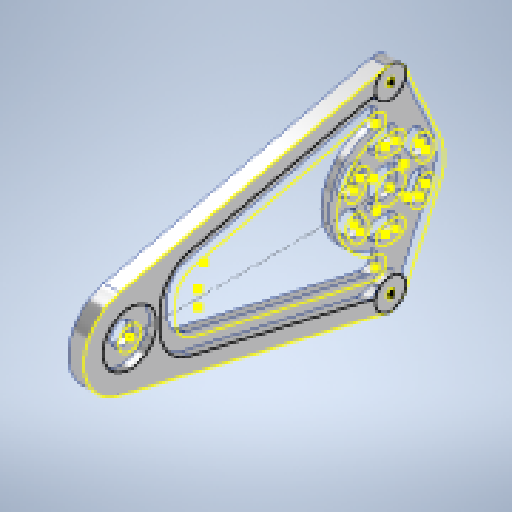
# Autodesk Inventor part: Frame (Motor Side)
Saved by Autodesk Inventor 2023.2 (Build 272271000, 271)
## iProperties
Created: 2022-05-22
Part Number: Frame (Motor Side)
Material: Aluminum 6061
Document SubType Name: Modeling
Designer: Nathan Cai
Density: 2.7 g/cm^3
Appearance: Aluminum - Flat
Mass: 77.655 g
Surface Area: 168.164 cm^2
Volume: 28.7611 cm^3
Author: Nathan Cai
Autodesk Inventor part; units mm, degrees
ref_plane "YZ Plane" through (0, 0, 0) normal (1, 0, 0) x (0, 1, 0)
ref_plane "XZ Plane" through (0, 0, 0) normal (0, 1, 0) x (-1, 0, 0)
ref_plane "XY Plane" through (0, 0, 0) normal (0, 0, 1) x (1, 0, 0)
sketch "Sketch1" plane through (0, 0, 0) normal (1, 0, 0) x (0, 1, 0)
  circle A0 centre (0, 0) radius 6
  circle A1 centre (0, 0) radius 22.225
  line L0 (0, 0) -> (0, 108.331) construction
  circle A2 centre (0, 108.331) radius 4.7625
  circle A3 centre (0, 108.331) radius 76.2 construction
  circle A4 centre (0, 108.331) radius 19.05
  line L1 (0, 0) -> (38.1, 0) construction
  circle A5 centre (38.1, 0) radius 1.7526
  arc A6 (31.9134, -1.4314) -> (35.4542, 5.7725) centre (38.1, 0) ccw
  line L2 (40.7458, -5.7725) -> (9.2604, -20.2038)
  line L3 (18.5597, 112.6252) -> (44.2866, 1.4314)
  line L4 (10.2351, 92.2641) -> (31.9134, -1.4314)
  line L5 (35.4542, 5.7725) -> (22.2231, -0.2919) construction
  circle A7 centre (-38.1, 0) radius 1.7526
  arc A8 (-35.4542, 5.7725) -> (-31.9134, -1.4314) centre (-38.1, 0) ccw
  line L6 (-40.7458, -5.7725) -> (-9.2604, -20.2038)
  line L7 (-18.5597, 112.6252) -> (-44.2866, 1.4314)
  line L8 (-10.2351, 92.2641) -> (-31.9134, -1.4314)
  line L9 (-35.4542, 5.7725) -> (-22.2231, -0.2919)
  line L10 (0, 0) -> (0, -9.5) construction
  line L11 (0, 0) -> (9.5, 0) construction
  line L12 (0, 0) -> (-8, 0) construction
  line L13 (0, 0) -> (-12.5, 0) construction
  line L14 (0, 0) -> (12.7, 0) construction
  line L15 (0, 0) -> (4.3437, -11.9341) construction
  line L16 (38.1, 0) -> (15.5738, 97.3602) construction
  circle A9 centre (19.05, 82.3358) radius 1.7526
  circle A10 centre (-19.05, 82.3358) radius 1.7526
  line L17 (-9, 9) -> (9, 9) construction
  circle A11 centre (5.6569, -5.6569) radius 1.5
  arc A12 (9.6641, 12.5945) -> (6.0751, 14.6666) centre (0, 0) ccw construction
  arc A13 (12.0991, 15.7679) -> (7.6058, 18.3621) centre (0, 0) ccw
  arc A14 (7.229, 9.4211) -> (4.5444, 10.9711) centre (0, 0) ccw
  arc A15 (7.229, 9.4211) -> (12.0991, 15.7679) centre (9.6641, 12.5945) ccw
  arc A16 (7.6058, 18.3621) -> (4.5444, 10.9711) centre (6.0751, 14.6666) ccw
  line L18 (0, 0) -> (6.0751, 14.6666) construction
  line L19 (0, 0) -> (9.6641, 12.5945) construction
  arc A17 (-4.5444, 10.9711) -> (-7.229, 9.4211) centre (0, 0) ccw
  arc A18 (-4.5444, 10.9711) -> (-7.6058, 18.3621) centre (-6.0751, 14.6666) ccw
  arc A19 (-12.0991, 15.7679) -> (-7.229, 9.4211) centre (-9.6641, 12.5945) ccw
  arc A20 (-6.0751, 14.6666) -> (-9.6641, 12.5945) centre (0, 0) ccw construction
  arc A21 (-7.6058, 18.3621) -> (-12.0991, 15.7679) centre (0, 0) ccw
  arc A22 (-11.7734, 1.55) -> (-11.7734, -1.55) centre (0, 0) ccw
  arc A23 (-11.7734, 1.55) -> (-19.705, 2.5942) centre (-15.7392, 2.0721) ccw
  arc A24 (-19.705, -2.5942) -> (-11.7734, -1.55) centre (-15.7392, -2.0721) ccw
  arc A25 (-15.7392, 2.0721) -> (-15.7392, -2.0721) centre (0, 0) ccw construction
  arc A26 (-19.705, 2.5942) -> (-19.705, -2.5942) centre (0, 0) ccw
  arc A27 (-7.229, -9.4211) -> (-4.5444, -10.9711) centre (0, 0) ccw
  arc A28 (-7.229, -9.4211) -> (-12.0991, -15.7679) centre (-9.6641, -12.5945) ccw
  arc A29 (-7.6058, -18.3621) -> (-4.5444, -10.9711) centre (-6.0751, -14.6666) ccw
  arc A30 (-9.6641, -12.5945) -> (-6.0751, -14.6666) centre (0, 0) ccw construction
  arc A31 (-12.0991, -15.7679) -> (-7.6058, -18.3621) centre (0, 0) ccw
  arc A32 (21.6386, 5.0715) -> (29.9605, 7.0094) centre (25.7982, 6.0464) ccw
  arc A33 (-29.9605, 7.0094) -> (-21.6386, 5.0715) centre (-25.7982, 6.0464) ccw
  line L20 (19.05, 82.3358) -> (-19.05, 82.3358) construction
  circle A34 centre (15.875, 82.3358) radius 6.35
  circle A35 centre (15.875, 82.3358) radius 1.7526
  circle A36 centre (-15.875, 82.3358) radius 6.35
  circle A37 centre (-15.875, 82.3358) radius 1.7526
  circle A38 centre (0, 0) radius 8 construction
  line L21 (5.6569, -5.6569) -> (0, 0) construction
  circle A39 centre (0, 0) radius 9.5 construction
  circle A40 centre (6.7175, 6.7175) radius 1.5
  line L22 (0, 0) -> (6.7175, 6.7175) construction
  arc A41 (4.5444, -10.9711) -> (7.229, -9.4211) centre (0, 0) ccw
  arc A42 (4.5444, -10.9711) -> (7.6058, -18.3621) centre (6.0751, -14.6666) ccw
  arc A43 (12.0991, -15.7679) -> (7.229, -9.4211) centre (9.6641, -12.5945) ccw
  arc A44 (6.0751, -14.6666) -> (9.6641, -12.5945) centre (0, 0) ccw construction
  arc A45 (7.6058, -18.3621) -> (12.0991, -15.7679) centre (0, 0) ccw
  arc A46 (11.7734, -1.55) -> (11.7734, 1.55) centre (0, 0) ccw
  arc A47 (11.7734, -1.55) -> (19.705, -2.5942) centre (15.7392, -2.0721) ccw
  arc A48 (19.705, 2.5942) -> (11.7734, 1.55) centre (15.7392, 2.0721) ccw
  arc A49 (15.7392, -2.0721) -> (15.7392, 2.0721) centre (0, 0) ccw construction
  arc A50 (19.705, -2.5942) -> (19.705, 2.5942) centre (0, 0) ccw
  circle A51 centre (-6.7175, -6.7175) radius 1.5
  circle A52 centre (-5.6569, 5.6569) radius 1.5
  point P0 (-18.5597, 112.6252)
  point P1 (-9.2604, -20.2038)
  point P2 (30.746, 3.6145)
  point P3 (-22.2231, -0.2919)
  point P4 (-30.746, 3.6145)
  point P5 (-21.6386, 5.0715)
  point P6 (-29.9605, 7.0094)
  point P7 (11.4733, 86.9126)
  point P8 (13.9309, 76.2907)
  point P9 (-13.9309, 76.2907)
  point P10 (-11.4733, 86.9126)
  dimension "d57" = 16
  dimension "d59" = 19
  dimension "d0" = 12
  dimension "d1" = 44.45
  dimension "d2" = 108.331
  dimension "d3" = 9.525
  dimension "d4" = 152.4
  dimension "d5" = 38.1
  dimension "d6" = 38.1
  dimension "d7" = 3.5052
  dimension "d8" = 12.7
  dimension "d9" = 0
  dimension "d10" = 12.7
  dimension "d11" = 12.7
  dimension "d15" = 9.5
  dimension "d16" = 270
  dimension "d18" = 8
  dimension "d35" = 70
  dimension "d36" = 3.5052
  dimension "d37" = 19.05
  dimension "d41" = 3
  dimension "d46" = 15.875
  dimension "d47" = 15
  dimension "d48" = 8
  dimension "d49" = 52.5
  dimension "d52" = 360
  dimension "d54" = 12.7
  dimension "d55" = 3.5052
  dimension "d56" = 15.875
  dimension "d58" = 45
  dimension "d60" = 3
  dimension "d67" = 360
  constraints: 78 point on circle, 51 centre point, 46 end point, 17 symmetric about line, 15 coincident, 11 tangent, 5 horizontal, 4 point on line, 3 parallel, 3 perpendicular, 1 collinear, 1 vertical, 94 other
  measures "d0" diameter of A0
  measures "d1" diameter of A1
  measures "d2" distance of L0.start L0.end
  measures "d3" diameter of A2
  measures "d4" diameter of A3
  measures "d5" diameter of A4
  measures "d6" distance of L1.start L1.end
  measures "d7" diameter of A5
  measures "d8" diameter of A6
  measures "d9" distance from line of A0.centre L1
  measures "d10" distance between parallel lines of L3 L4
  measures "d11" distance between parallel lines of L2 L5
  measures "d15" distance of L0.start L10.end
  measures "d18" distance of L0.start L12.end
  measures "d35" angle of L11 L15
  measures "d36" diameter of A9
  measures "d37" distance from line of L0 L20.start
  measures "d41" diameter of A11
  measures "d46" radius of A12
  measures "d47" angle of L19 L18
  measures "d48" diameter of A16
  measures "d49" angle of L11 L19
  measures "d54" diameter of A34
  measures "d55" diameter of A35
  measures "d56" distance from line of L0 A35.centre
  measures "d58" angle of L21 L1
  measures "d60" diameter of A40
extrude "Extrusion1" add sketch "Sketch1" along normal blind 6.35 contours A1 | A1 A32 L4 A6 L2 | A1 L9 A33 | L4 A34 A4 L3 A6 | L6 A8 L8 L9 A1 | L9 L8 A33 | L4 A34 | A8 L9 L8 | L9 A8 L7 A4 L8 A36 | A4 | A36 L8 | A9 A35 | A35 A9 | A9 A35 | A10 A37 | A10 A37 | A37 A10 picked at (13.1931, 81.7042) picked at (-13.1931, 81.7042)
fillet "Fillet1" radius 9.525 2 edges at (3.175, 10.2351, 92.2641) (3.175, -10.2351, 92.2641)
sketch "Sketch2" plane through (6.35, 0, 0) normal (1, 0, 0) x (0, 0, -1)
  arc A0 (5.7725, 40.7458) -> (-1.4314, 44.2866) centre (0, 38.1) ccw projected
  line L0 (-1.4314, 44.2866) -> (-112.6252, 18.5597) projected
  arc A1 (-112.6252, 18.5597) -> (-112.6252, -18.5597) centre (-108.331, 0) ccw projected
  line L1 (-112.6252, -18.5597) -> (-1.4314, -44.2866) projected
  arc A2 (-1.4314, -44.2866) -> (5.7725, -40.7458) centre (0, -38.1) ccw projected
  line L2 (5.7725, -40.7458) -> (20.2038, -9.2604) projected
  arc A3 (20.2038, -9.2604) -> (20.2038, 9.2604) centre (0, 0) ccw projected
  line L3 (20.2038, 9.2604) -> (5.7725, 40.7458) projected
  arc A4 (-5.0715, 21.6386) -> (-5.0715, -21.6386) centre (0, 0) ccw projected
  arc A5 (-7.0094, -29.9605) -> (-5.0715, -21.6386) centre (-6.0464, -25.7982) ccw projected
  line L4 (-7.0094, -29.9605) -> (-82.0952, -12.5879) projected
  arc A6 (-89.4091, -2.2054) -> (-89.4091, 2.2054) centre (-108.331, 0) ccw projected
  line L5 (-82.0952, 12.5879) -> (-7.0094, 29.9605) projected
  arc A7 (-5.0715, 21.6386) -> (-7.0094, 29.9605) centre (-6.0464, 25.7982) ccw projected
  circle A8 centre (0, 0) radius 6 projected
  circle A9 centre (5.6569, 5.6569) radius 1.5 projected
  arc A10 (-9.4211, 7.229) -> (-10.9711, 4.5444) centre (0, 0) ccw projected
  arc A11 (-18.3621, 7.6058) -> (-10.9711, 4.5444) centre (-14.6666, 6.0751) ccw projected
  arc A12 (-15.7679, 12.0991) -> (-18.3621, 7.6058) centre (0, 0) ccw projected
  arc A13 (-9.4211, 7.229) -> (-15.7679, 12.0991) centre (-12.5945, 9.6641) ccw projected
  arc A14 (-10.9711, -4.5444) -> (-18.3621, -7.6058) centre (-14.6666, -6.0751) ccw projected
  arc A15 (-10.9711, -4.5444) -> (-9.4211, -7.229) centre (0, 0) ccw projected
  arc A16 (-15.7679, -12.0991) -> (-9.4211, -7.229) centre (-12.5945, -9.6641) ccw projected
  arc A17 (-18.3621, -7.6058) -> (-15.7679, -12.0991) centre (0, 0) ccw projected
  arc A18 (-1.55, -11.7734) -> (-2.5942, -19.705) centre (-2.0721, -15.7392) ccw projected
  arc A19 (-1.55, -11.7734) -> (1.55, -11.7734) centre (0, 0) ccw projected
  arc A20 (2.5942, -19.705) -> (1.55, -11.7734) centre (2.0721, -15.7392) ccw projected
  arc A21 (-2.5942, -19.705) -> (2.5942, -19.705) centre (0, 0) ccw projected
  arc A22 (9.4211, -7.229) -> (15.7679, -12.0991) centre (12.5945, -9.6641) ccw projected
  arc A23 (9.4211, -7.229) -> (10.9711, -4.5444) centre (0, 0) ccw projected
  arc A24 (18.3621, -7.6058) -> (10.9711, -4.5444) centre (14.6666, -6.0751) ccw projected
  arc A25 (15.7679, -12.0991) -> (18.3621, -7.6058) centre (0, 0) ccw projected
  circle A26 centre (-6.7175, 6.7175) radius 1.5 projected
  arc A27 (10.9711, 4.5444) -> (18.3621, 7.6058) centre (14.6666, 6.0751) ccw projected
  arc A28 (10.9711, 4.5444) -> (9.4211, 7.229) centre (0, 0) ccw projected
  arc A29 (15.7679, 12.0991) -> (9.4211, 7.229) centre (12.5945, 9.6641) ccw projected
  arc A30 (18.3621, 7.6058) -> (15.7679, 12.0991) centre (0, 0) ccw projected
  arc A31 (1.55, 11.7734) -> (2.5942, 19.705) centre (2.0721, 15.7392) ccw projected
  arc A32 (1.55, 11.7734) -> (-1.55, 11.7734) centre (0, 0) ccw projected
  arc A33 (-2.5942, 19.705) -> (-1.55, 11.7734) centre (-2.0721, 15.7392) ccw projected
  arc A34 (2.5942, 19.705) -> (-2.5942, 19.705) centre (0, 0) ccw projected
  circle A35 centre (6.7175, -6.7175) radius 1.5 projected
  circle A36 centre (-5.6569, -5.6569) radius 1.5 projected
  circle A37 centre (0, 38.1) radius 1.7526 projected
  circle A38 centre (0, -38.1) radius 1.7526 projected
  circle A39 centre (-108.331, 0) radius 4.7625 projected
  circle A40 centre (-108.331, 0) radius 11.1125
  arc A41 (5.7725, 40.7458) -> (-1.4314, 44.2866) centre (0, 38.1) ccw projected
  circle A42 centre (0, 38.1) radius 6.35
  circle A43 centre (0, -38.1) radius 1.7526 projected
  arc A44 (-1.4314, -44.2866) -> (5.7725, -40.7458) centre (0, -38.1) ccw projected
  circle A45 centre (0, -38.1) radius 6.35
  line L6 (-108.331, 0) -> (0, 0) construction
  arc A46 (-5.0715, 21.6386) -> (-7.0094, 29.9605) centre (-6.0464, 25.7982) ccw projected
  arc A47 (-89.4091, -2.2054) -> (-82.0952, -12.5879) centre (-79.9481, -3.3081) ccw projected
  arc A48 (-82.0952, 12.5879) -> (-89.4091, 2.2054) centre (-79.9481, 3.3081) ccw projected
  line L7 (-6.1866, 36.6686) -> (-83.5266, 18.7745)
  arc A49 (-83.5266, 18.7745) -> (-95.7164, 1.4702) centre (-79.9481, 3.3081) ccw
  arc A50 (-95.7164, -1.4702) -> (-95.7164, 1.4702) centre (-108.331, 0) ccw
  arc A51 (-95.7164, -1.4702) -> (-83.5266, -18.7745) centre (-79.9481, -3.3081) ccw
  line L8 (-83.5266, -18.7745) -> (-6.1866, -36.6686)
  point P0 (-77.5142, 11.7428)
  point P1 (5.7725, 40.7458)
  dimension "d69" = 22.225
  dimension "d77" = 6.35
  dimension "d78" = 6.35
  constraints: 10 point on circle, 6 centre point, 6 end point, 3 coincident, 1 horizontal, 3 other
  measures "d69" diameter of A40
  measures "d77" distance between parallel lines of L5 L7
  measures "d78" radial gap between concentric circles of A48 A49
extrude "Extrusion2" cut sketch "Sketch2" against normal blind 3.175 contours L3 A3 L2 A45 L8 A51 A50 A49 L7 A42
extrude "Extrusion3" cut sketch "Sketch2" against normal blind 3.175 contours A40
fillet "Fillet2" radius 6.35 2 edges at (4.7625, 36.6686, 6.1866) (4.7625, -36.6686, 6.1866)
equation "\"d10\" = d8"
equation "\"d11\" = d10"
equation "\"Leg_Mounts\" = 15.875"
equation "\"Leg_Offset\" = 19.05"
equation "\"C2C\" = 107.95"
body "Solid1"
